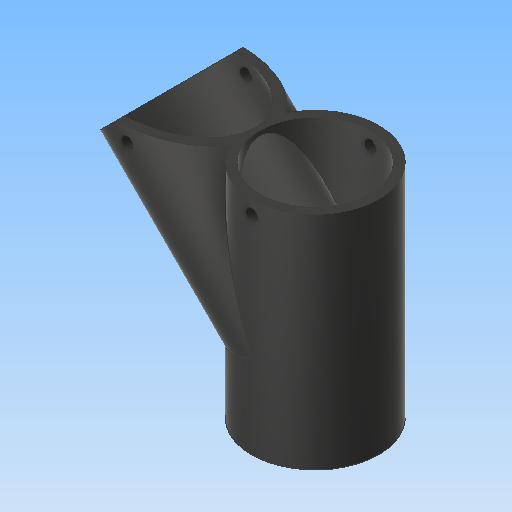
# Autodesk Inventor part: Top_45 Deg Connector
Saved by Autodesk Inventor 2018.1 (Build 221171000, 171)
## iProperties
Created: 2019-03-22
Part Number: Top_45 Deg Connector
Material: PVC-Piping
Document SubType Name: Modeling
Designer: James
Density: 1.4 g/cm^3
Appearance: Smooth - Black
Author: James
Autodesk Inventor part; units mm, degrees
ref_plane "YZ Plane" through (0, 0, 0) normal (1, 0, 0) x (0, 1, 0)
sketch "Sketch1" plane through (0, 0, 0) normal (0, 1, 0) x (-1, 0, 0)
  circle A0 centre (0, 0) radius 20
  circle A1 centre (0, 0) radius 23
  dimension "d0" = 40
  dimension "d1" = 46
  constraints: 2 centre point, 2 coincident
  measures "d0" diameter of A0
  measures "d1" diameter of A1
extrude "Extrusion1" add sketch "Sketch1" along normal mid plane 140
ref_plane "Work Plane1" through (0, 0, 0) normal (-0.7071068, 0.7071068, 0) x (0, 0, 1)
sketch "Sketch2" plane through (0, 0, 0) normal (-0.7071068, 0.7071068, 0) x (0, 0, 1)
  circle A0 centre (0, 0) radius 20
  circle A1 centre (0, 0) radius 23
  dimension "d5" = 40
  dimension "d6" = 46
  constraints: 2 centre point, 2 coincident
  measures "d5" diameter of A0
  measures "d6" diameter of A1
extrude "Extrusion2" add sketch "Sketch2" along normal blind 70
sketch "Sketch3" plane through (0, 70, 0) normal (0, 1, 0) x (1, 0, 0)
  circle A0 centre (0, 0) radius 20 projected
extrude "Extrusion3" cut sketch "Sketch3" against normal through all
sketch "Sketch4" plane through (-49.4975, 49.4975, 0) normal (-0.7071068, 0.7071068, 0) x (-0.7071068, -0.7071068, 0)
  circle A0 centre (0, 0) radius 20 projected
extrude "Extrusion4" cut sketch "Sketch4" against normal up to next
sketch "Sketch5" plane through (0, -70, 0) normal (0, -1, 0) x (1, 0, 0)
  circle A0 centre (0, 0) radius 20 projected
  circle A1 centre (0, 0) radius 23 projected
extrude "Extrusion5" cut sketch "Sketch5" against normal blind 40
sketch "Sketch6" plane through (0, 0, 0) normal (0, 0, 1) x (1, 0, 0)
  line L0 (23, 70) -> (-97, 70)
  line L1 (-97, 70) -> (-97, 50)
  line L2 (-97, 50) -> (23, 50)
  line L3 (23, 50) -> (23, 70)
  line L4 (23, -30) -> (-23, -30) projected
  line L5 (0, 0) -> (0, 0) projected
  line L6 (0, 0) -> (0, 0) projected
  line L7 (23, 70) -> (-23, 70) projected
  dimension "d15" = 120
  dimension "d16" = 20
  constraints: 8 end point, 2 coincident, 2 parallel, 1 horizontal, 1 perpendicular
  measures "d15" distance of L0.start L0.end
  measures "d16" distance of L0.end L1.end
extrude "Extrusion6" cut sketch "Sketch6" along normal through all both and the other way through all
ref_plane "Work Plane2" through (0, 0, 50) normal (0, 0, 1) x (1, 0, 0)
sketch "Sketch7" plane through (0, 0, 50) normal (0, 0, 1) x (1, 0, 0)
  line L0 (-20.7107, 50) -> (23, 50) projected
  line L1 (20, 50) -> (-20, 50) projected
  point P0 (0, 0)
  point P1 (-45, 45)
  point P2 (0, 45)
  dimension "d20" = 5
  dimension "d21" = 45
  constraints: 1 horizontal alignment, 1 vertical alignment
  measures "d20" distance from line of L0 point (0, 45)
  measures "d21" distance of point (0, 45) point (-45, 45)
hole "Hole1" at (-45, 45, 50) at (0, 45, 50) direction (0, 0, -1) diameter 4.5 end through all clearance for "Flat Head Machine Screw" size "M4" standard "Ansi Metric M Profile"
body "Solid1"
